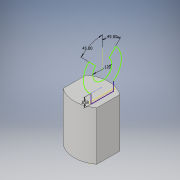
# Autodesk Inventor part: Hand-y doo dad
Saved by Autodesk Inventor 2017 (Build 210142000, 142)
## iProperties
Created: 2018-05-14
Part Number: Hand-y doo dad
Material: Generic
Document SubType Name: Modeling
Designer: Kyle
Density: 1 g/cm^3
Appearance: Default
Author: Kyle
Autodesk Inventor part; units mm, degrees
ref_plane "YZ Plane" through (0, 0, 0) normal (1, 0, 0) x (0, 1, 0)
ref_plane "XZ Plane" through (0, 0, 0) normal (0, 1, 0) x (-1, 0, 0)
ref_plane "XY Plane" through (0, 0, 0) normal (0, 0, 1) x (1, 0, 0)
sketch "Sketch1" plane through (0, 0, 0) normal (0, 1, 0) x (-1, 0, 0)
  line L0 (0, 0) -> (2.6987, 0) construction
  line L1 (2.6987, 0) -> (2.6987, -2.7407) construction
  line L2 (2.6987, -2.7407) -> (0, -2.7407) construction
  line L3 (0, -2.7407) -> (0, 0) construction
  line L4 (2.6987, 0) -> (2.6987, -1.8263) construction
  line L5 (2.6987, 0) -> (4.525, 0) construction
  arc A0 (0, -2.7407) -> (2.6987, -1.8263) centre (0, 1.6991) ccw
  line L6 (2.6987, -1.8263) -> (2.6987, 0)
  arc A1 (-2.6987, -1.8263) -> (0, -2.7407) centre (0, 1.6991) ccw
  line L7 (-2.6987, -1.8263) -> (-2.6987, 0)
  arc A2 (2.6987, 1.8263) -> (0, 2.7407) centre (0, -1.6991) ccw
  line L8 (2.6987, 1.8263) -> (2.6987, 0)
  arc A3 (0, 2.7407) -> (-2.6987, 1.8263) centre (0, -1.6991) ccw
  line L9 (-2.6987, 1.8263) -> (-2.6987, 0)
  dimension "d0" = 2.6987
  dimension "d1" = 2.7407
  dimension "d2" = 1.8263
  dimension "d3" = 90
  constraints: 20 end point, 8 point on circle, 6 symmetric about line, 4 centre point, 2 collinear, 2 horizontal, 2 parallel, 2 perpendicular, 1 tangent, 3 other
  measures "d0" distance of L1.end L2.end
  measures "d1" distance of L0.end L1.end
  measures "d2" distance of L0.end L4.end
  measures "d3" angle of L4 L5
extrude "Extrusion1" add sketch "Sketch1" along normal blind 7.8334
sketch "Sketch2" plane through (0, 0, 0) normal (0, -1, 0) x (1, 0, 0)
  circle A0 centre (0, 0) radius 1.5862
  dimension "d6" = 3.1725
  constraints: 1 centre point, 1 coincident
  measures "d6" diameter of A0
extrude "Extrusion2" cut sketch "Sketch2" against normal blind 4.0589
ref_plane "Work Plane1" through (1.7107, 0, 1.8263) normal (1, 0, 0) x (0, 0, -1)
sketch "Sketch3" plane through (1.7107, 0, 1.8263) normal (1, 0, 0) x (0, 0, -1)
  line L0 (3.6525, 7.8334) -> (0, 7.8334) projected
  line L1 (3.6525, 7.8334) -> (0, 7.8334)
  line L2 (0, 7.8334) -> (0, 9.3066)
  line L3 (0, 9.3066) -> (1.8263, 9.3066) construction
  line L4 (3.6525, 9.3066) -> (3.6525, 7.8334)
  arc A0 (0.7459, 12.8145) -> (2.9066, 12.8145) centre (1.8263, 11.7342) ccw
  line L5 (1.8263, 11.7342) -> (1.8263, 14.772) construction
  line L6 (2.9066, 12.8145) -> (3.9743, 13.8822)
  line L7 (0.7459, 12.8145) -> (-0.3218, 13.8822)
  arc A1 (-0.3218, 13.8822) -> (0, 9.3066) centre (1.8263, 11.7342) ccw
  arc A2 (3.6525, 9.3066) -> (3.9743, 13.8822) centre (1.8263, 11.7342) ccw
  point P0 (1.8263, 0)
  dimension "d10" = 1.4732
  dimension "d12" = 3.0556
  dimension "d13" = 45
  dimension "d14" = 45
  constraints: 14 end point, 6 point on circle, 3 centre point, 2 parallel, 2 vertical, 1 coincident, 1 horizontal, 1 perpendicular, 1 point on line
  measures "d10" distance of L1.end L2.end
  measures "d12" diameter of A0
body "Solid1"
